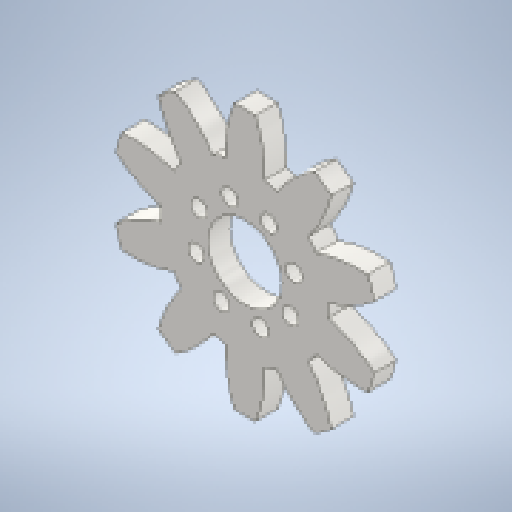
# Autodesk Inventor part: 平歯車1
Saved by Autodesk Inventor 2024 (Build 280153000, 153)
## iProperties
Created: 2024-06-05
Part Number: 平歯車1
Material: Steel
Document SubType Name: Modeling
Designer: right
Categories: <?xml version="1.0" encoding="UTF-16"?> <MemberInstance><Categories><FamilyTemplate><FamilyTemplateParameter ValueType="xs:double" Id="1" ObjectReferenceKey="da_z" ObjectType="kUserParameterObject"/><FamilyTemplateParameter ValueType="xs:double" Id="2" ObjectReferenceKey="da_b" ObjectType="kUserParameterObject"/><FamilyTemplateParameter ValueType="xs:double" Id="3" ObjectReferenceKey="da_beta" ObjectType="kUserParameterObject"/><FamilyTemplateParameter ValueType="xs:double" Id="4" ObjectReferenceKey="da_da" ObjectType="kUserParameterObject"/><FamilyTemplateParameter ValueType="xs:double" Id="5" ObjectReferenceKey="da_aw" ObjectType="kUserParameterObject"/><FamilyTemplateParameter ValueType="xs:string" Id="6" ObjectReferenceKey="EAIAABAAAACIAQAAAAAAAIAAAAAAAAAA" ObjectType="83910656" SubObjectId="SurfaceGeometry"/></FamilyTemplate><ParamToTemplateMap><ParamToTemplate CategoryParameter="//CategoryParameter[@InternalName='046C89C9-8512-4d59-83FE-43B91F4F132A']" TemplateParameter="1"/><ParamToTemplate CategoryParameter="//CategoryParameter[@InternalName='2552DF32-E462-4b46-AEBF-C6C7768E72AC']" TemplateParameter="2"/><ParamToTemplate CategoryParameter="//CategoryParameter[@InternalName='C9EE641D-15FC-4fae-A226-E94C4372FDD7']" TemplateParameter="3"/><ParamToTemplate><ParamToTemplate CategoryParameter="//CategoryParameter[@InternalName='00B6519A-459B-49c7-AD84-2E56D39A5744']" ConstantValue="0.035417"/></ParamToTemplate><ParamToTemplate><ParamToTemplate CategoryParameter="//CategoryParameter[@InternalName='04B31F0E-C7A6-4894-AA32-9629BEFACF47']" ConstantValue="1.000000"/></ParamToTemplate><ParamToTemplate><ParamToTemplate CategoryParameter="//CategoryParameter[@InternalName='43CBEC2E-7847-49e7-A936-2F7889FCB2D9']" ConstantValue="0.250000"/></ParamToTemplate><ParamToTemplate><ParamToTemplate CategoryParameter="//CategoryParameter[@InternalName='B1EFC894-105D-4ebd-86BF-FA20ED196853']" ConstantValue="0.350000"/></ParamToTemplate><ParamToTemplate><ParamToTemplate CategoryParameter="//CategoryParameter[@InternalName='51175063-3D10-4879-93E8-6246FE8B403D']" ConstantValue="2060000000.000000"/></ParamToTemplate><ParamToTemplate><ParamToTemplate CategoryParameter="//CategoryParameter[@InternalName='A3A52E27-4454-46a9-B0BD-C932399B70AF']" ConstantValue="0.300000"/></ParamToTemplate><ParamToTemplate><ParamToTemplate CategoryParameter="//CategoryParameter[@InternalName='91B76062-C214-41d9-B1B9-14D2AB99603D']" ConstantValue="0.300000"/></ParamToTemplate><ParamToTemplate><ParamToTemplate CategoryParameter="//CategoryParameter[@InternalName='374E806E-8B8A-4dda-A9AA-1039D6500AD2']" ConstantValue="3.333333"/></ParamToTemplate><ParamToTemplate><ParamToTemplate CategoryParameter="//CategoryParameter[@InternalName='2D373A89-B862-43d6-8D0B-0CBF12AB9F6C']" ConstantValue="0.349066"/></ParamToTemplate><ParamToTemplate CategoryParameter="//CategoryParameter[@InternalName='37777632-D6A2-4fac-9D53-DB8ACD95C989']" TemplateParameter="4"/><ParamToTemplate CategoryParameter="//CategoryParameter[@InternalName='FD1017F1-B727-4f7e-9707-0F86F1FF9423']" TemplateParameter="5"/><ParamToTemplate><ParamToTemplate CategoryParameter="//CategoryParameter[@InternalName='9E1B4470-B2D3-4ff1-B813-535BB4CDF51A']" ConstantValue="3520000.000000"/></ParamToTemplate><ParamToTemplate><ParamToTemplate CategoryParameter="//CategoryParameter[@InternalName='F8452263-BFF6-458c-9FB1-07C4B99E95CD']" ConstantValue="11400000.000000"/></ParamToTemplate><ParamToTemplate><ParamToTemplate CategoryParameter="//CategoryParameter[@InternalName='3E3BB259-FD49-497f-8171-6EBC954A3479']" ConstantValue="2.000000"/></ParamToTemplate><ParamToTemplate CategoryParameter="//CategoryParameter[@InternalName='27C3BAF2-7550-4e4b-AE2C-0DB134B7D9B7']" TemplateParameter="6"/></ParamToTemplateMap><Category DisplayName="Gear" InternalName="DC85795E-93AB-48d5-8EEE-5A27447B64BD" Mnemonic="Gear"><CategoryParameter DisplayName="z" InternalName="046C89C9-8512-4d59-83FE-43B91F4F132A" Mnemonic="z"/><CategoryParameter DisplayName="b" InternalName="2552DF32-E462-4b46-AEBF-C6C7768E72AC" Mnemonic="b"/><CategoryParameter DisplayName="||b|" InternalName="C9EE641D-15FC-4fae-A226-E94C4372FDD7" Mnemonic="beta"/><CategoryParameter DisplayName="x" InternalName="00B6519A-459B-49c7-AD84-2E56D39A5744" Mnemonic="x"/><CategoryParameter DisplayName="a*" InternalName="04B31F0E-C7A6-4894-AA32-9629BEFACF47" Mnemonic="a"/><CategoryParameter DisplayName="c*" InternalName="43CBEC2E-7847-49e7-A936-2F7889FCB2D9" Mnemonic="c"/><CategoryParameter DisplayName="r|.f|*" InternalName="B1EFC894-105D-4ebd-86BF-FA20ED196853" Mnemonic="rf"/><CategoryParameter DisplayName="E" InternalName="51175063-3D10-4879-93E8-6246FE8B403D" Mnemonic="E"/><CategoryParameter DisplayName="||m|" InternalName="A3A52E27-4454-46a9-B0BD-C932399B70AF" Mnemonic="mi"/><Category DisplayName="SpurGear" InternalName="26C5A22E-A91E-4dfd-A3B3-23CCAFAE1764" Mnemonic="SpurGear"><CategoryParameter DisplayName="m" InternalName="91B76062-C214-41d9-B1B9-14D2AB99603D" Mnemonic="m"/><CategoryParameter DisplayName="P" InternalName="374E806E-8B8A-4dda-A9AA-1039D6500AD2" Mnemonic="PP"/><CategoryParameter DisplayName="||a|" InternalName="2D373A89-B862-43d6-8D0B-0CBF12AB9F6C" Mnemonic="alpha"/><CategoryParameter DisplayName="d|.a|" InternalName="37777632-D6A2-4fac-9D53-DB8ACD95C989" Mnemonic="da"/><CategoryParameter DisplayName="a|.w|" InternalName="FD1017F1-B727-4f7e-9707-0F86F1FF9423" Mnemonic="aw"/><CategoryParameter DisplayName="||s||.Flim|" InternalName="9E1B4470-B2D3-4ff1-B813-535BB4CDF51A" Mnemonic="sFlim"/><CategoryParameter DisplayName="||s||.Hlim|" InternalName="F8452263-BFF6-458c-9FB1-07C4B99E95CD" Mnemonic="sHlim"/><CategoryParameter DisplayName="タイプ" InternalName="3E3BB259-FD49-497f-8171-6EBC954A3479" Mnemonic="type"/><CategoryParameter DisplayName="PitchDiameter" InternalName="27C3BAF2-7550-4e4b-AE2C-0DB134B7D9B7" Mnemonic="IDS_PITCHDIAM"/></Category></Category></Categories></MemberInstance>
Density: 1 g/cm^3
Appearance: Steel
CustomPartVersion: 1
Author: right
Autodesk Inventor part; units mm, degrees
ref_plane "YZ Plane" through (0, 0, 0) normal (1, 0, 0) x (0, 1, 0)
ref_plane "XZ Plane" through (0, 0, 0) normal (0, 1, 0) x (-1, 0, 0)
ref_plane "XY Plane" through (0, 0, 0) normal (0, 0, 1) x (1, 0, 0)
sketch "Sketch1" plane through (0, 0, 0) normal (0, 0, 1) x (1, 0, 0)
  circle A0 centre (0, 0) radius 18.1063
  dimension "d0" = 36.2125
  constraints: 1 centre point
  measures "d0" diameter of A0
extrude "Extrusion1" add sketch "Sketch1" along normal blind 30
ref_plane "Work Plane2" through (0, 0, 15) normal (0, 0, 1) x (1, 0, 0)
sketch "Sketch2" plane through (0, 0, 0) normal (0, 0, -1) x (-1, 0, 0)
  circle A0 centre (0, 0) radius 18.1063 projected
  circle A1 centre (0, 0) radius 15
  dimension "d3" = 30
  constraints: 1 centre point, 1 coincident
  measures "d3" diameter of A1
surface extrude "ピッチ円直径" sketch "Sketch2" against normal through all shown no curves A1
ref_plane "Work Plane8" through (0, 0, 0) normal (0.9510565, 0.309017, 0) x (0, 0, 1)
ref_plane "Work Plane9" through (0, 0, 0) normal (1, 0, 0) x (0, 1, 0)
spur gear teeth "平歯車" teeth 10 pitch diameter 30 tip diameter 36.2125 root diameter 22.7125 face width 30 start plane through (0, 0, 0) normal (0, 0, -1) x (-1, 0, 0)
sketch "スケッチ3" plane through (0, 0, 30) normal (0, 0, 1) x (1, 0, 0)
  arc A0 (-11.7591, 13.7681) -> (-8.6354, 7.3753) centre (4.2073, 17.6101) ccw projected
  arc A1 (-8.6354, 7.3753) -> (-9.6828, 5.9336) centre (0, 0) ccw projected
  arc A2 (-9.6828, 5.9336) -> (-16.728, 6.929) centre (-15.4481, -9.4432) ccw projected
  arc A3 (-16.728, 6.929) -> (-17.606, 4.2268) centre (0, 0) ccw projected
  arc A4 (-17.606, 4.2268) -> (-11.3212, 0.891) centre (-6.9472, 16.7199) ccw projected
  arc A5 (-11.3212, 0.891) -> (-11.3212, -0.891) centre (0, 0) ccw projected
  arc A6 (-11.3212, -0.891) -> (-17.606, -4.2268) centre (-6.9472, -16.7199) ccw projected
  arc A7 (-17.606, -4.2268) -> (-16.728, -6.929) centre (0, 0) ccw projected
  arc A8 (-16.728, -6.929) -> (-9.6828, -5.9336) centre (-15.4481, 9.4432) ccw projected
  arc A9 (-9.6828, -5.9336) -> (-8.6354, -7.3753) centre (0, 0) ccw projected
  arc A10 (-8.6354, -7.3753) -> (-11.7591, -13.7681) centre (4.2073, -17.6101) ccw projected
  arc A11 (-11.7591, -13.7681) -> (-9.4605, -15.4381) centre (0, 0) ccw projected
  arc A12 (-9.4605, -15.4381) -> (-4.3458, -10.4918) centre (-18.0484, -1.4405) ccw projected
  arc A13 (-4.3458, -10.4918) -> (-2.6511, -11.0425) centre (0, 0) ccw projected
  arc A14 (-2.6511, -11.0425) -> (-1.4206, -18.0504) centre (13.7548, -11.7739) ccw projected
  arc A15 (-1.4206, -18.0504) -> (1.4206, -18.0504) centre (0, 0) ccw projected
  arc A16 (1.4206, -18.0504) -> (2.6511, -11.0425) centre (-13.7548, -11.7739) ccw projected
  arc A17 (2.6511, -11.0425) -> (4.3458, -10.4918) centre (0, 0) ccw projected
  arc A18 (4.3458, -10.4918) -> (9.4605, -15.4381) centre (18.0484, -1.4405) ccw projected
  arc A19 (9.4605, -15.4381) -> (11.7591, -13.7681) centre (0, 0) ccw projected
  arc A20 (11.7591, -13.7681) -> (8.6354, -7.3753) centre (-4.2073, -17.6101) ccw projected
  arc A21 (8.6354, -7.3753) -> (9.6828, -5.9336) centre (0, 0) ccw projected
  arc A22 (9.6828, -5.9336) -> (16.728, -6.929) centre (15.4481, 9.4432) ccw projected
  arc A23 (16.728, -6.929) -> (17.606, -4.2268) centre (0, 0) ccw projected
  arc A24 (17.606, -4.2268) -> (11.3212, -0.891) centre (6.9472, -16.7199) ccw projected
  arc A25 (11.3212, -0.891) -> (11.3212, 0.891) centre (0, 0) ccw projected
  arc A26 (11.3212, 0.891) -> (17.606, 4.2268) centre (6.9472, 16.7199) ccw projected
  arc A27 (17.606, 4.2268) -> (16.728, 6.929) centre (0, 0) ccw projected
  arc A28 (16.728, 6.929) -> (9.6828, 5.9336) centre (15.4481, -9.4432) ccw projected
  arc A29 (9.6828, 5.9336) -> (8.6354, 7.3753) centre (0, 0) ccw projected
  arc A30 (8.6354, 7.3753) -> (11.7591, 13.7681) centre (-4.2073, 17.6101) ccw projected
  arc A31 (11.7591, 13.7681) -> (9.4605, 15.4381) centre (0, 0) ccw projected
  arc A32 (9.4605, 15.4381) -> (4.3458, 10.4918) centre (18.0484, 1.4405) ccw projected
  arc A33 (4.3458, 10.4918) -> (2.6511, 11.0425) centre (0, 0) ccw projected
  arc A34 (2.6511, 11.0425) -> (1.4206, 18.0504) centre (-13.7548, 11.7739) ccw projected
  arc A35 (1.4206, 18.0504) -> (-1.4206, 18.0504) centre (0, 0) ccw projected
  arc A36 (-1.4206, 18.0504) -> (-2.6511, 11.0425) centre (13.7548, 11.7739) ccw projected
  arc A37 (-2.6511, 11.0425) -> (-4.3458, 10.4918) centre (0, 0) ccw projected
  arc A38 (-4.3458, 10.4918) -> (-9.4605, 15.4381) centre (-18.0484, 1.4405) ccw projected
  arc A39 (-9.4605, 15.4381) -> (-11.7591, 13.7681) centre (0, 0) ccw projected
ref_plane "作業平面11" through (-21.9768, -21.9768, 3) normal (0, 0, 1) x (0.9530718, 0.3027442, 0)
extrude "押し出し2" cut sketch "スケッチ3" against normal up to surface (27 mm away)
sketch "スケッチ4" plane through (0, 0, 3) normal (0, 0, 1) x (1, 0, 0)
  circle A0 centre (0, 0) radius 17.5 projected
  circle A1 centre (0, 0) radius 5 projected
  circle A2 centre (-2.1192, 6.6715) radius 1.1 projected
  circle A3 centre (-6.216, 3.219) radius 1.1 projected
  circle A4 centre (-6.6715, -2.1192) radius 1.1 projected
  circle A5 centre (-3.219, -6.216) radius 1.1 projected
  circle A6 centre (2.1192, -6.6715) radius 1.1 projected
  circle A7 centre (6.216, -3.219) radius 1.1 projected
  circle A8 centre (6.6715, 2.1192) radius 1.1 projected
  circle A9 centre (3.219, 6.216) radius 1.1 projected
  point P0 (0, 0)
extrude "押し出し3" cut sketch "スケッチ4" against normal through all contours A1 | A2 | A3 | A4 | A5 | A6 | A7 | A8 | A9
sketch "スケッチ5" plane through (0, 0, 3) normal (0, 0, 1) x (1, 0, 0)
  circle A0 centre (0, 0) radius 10
  circle A1 centre (-6.6715, -2.1192) radius 1.1 construction
  circle A2 centre (-6.6715, -2.1192) radius 3 construction
  dimension "d53" = 6
  constraints: 2 centre point, 2 coincident, 1 tangent
  measures "d53" diameter of A2
extrude "押し出し4" cut sketch "スケッチ5" against normal blind 1.5
equation "\"d0\" = da_da"
equation "\"d1\" = da_b"
equation "\"d3\" = da_d"
equation "\"da_da\" = 36.2125"
equation "\"da_b\" = 30"
equation "\"da_d\" = 30"
body "Solid1"
body "Srf1"
